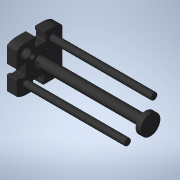
# Autodesk Inventor part: 537123 ADNGF-12-40-P-A---(KS)
Saved by Autodesk Inventor 2021 (Build 250183000, 183)
## iProperties
Created: 2025-06-05
Part Number: 537123 ADNGF-12-40-P-A---(KS)
Material: Generic
Catalog Web Link: www.cadenas.de
Description: ADNGF-(KS)-Compact cylinder - piston rod
Vendor: FESTO
Document SubType Name: Modeling
Designer: psAdmin
Manufacturer: FESTO
Mass: 6.99513 g
Surface Area: 56.7933 cm^2
Volume: 6.99513 cm^3
Density: 1 g/cm^3
Appearance: PSOLRGB-175-175-175
Category: PARTsolutions
Company: FESTO
Title: 537123 ADNGF-12-40-P-A---(KS)
Author: Cadenas PARTsolutions
Comments: Compact cylinder - piston rod
PSOL_IDENT_0: {$CADENAS_DATA/23d-libs/festo/parts/a/adngf/parts/adngf_ks.prj},219 {VTYP=3D},{NB=537123 ADNGF-12-40
PSOL_IDENT_1: -P-A---(KS)},{LINA=537123 ADNGF-12-40-P-A---(KS)},{NN=ADNGF-(KS)},{DATE=02.05.2022 12:53:58},{GEOMDA
PSOL_IDENT_2: TE=02.05.2022 12:53:00},{VERSION=},{LINEID=5510},{WBVAR=HUB,DF,S2S20},{WBNUMERIC=HUB}  {NB=537123 AD
PSOL_IDENT_3: NGF-12-40-P-A---(KS)},{LINA=537123 ADNGF-12-40-P-A---(KS)},{KT=ADNGF-12},{TNR=537123},{AUSF=ADNGF-12
PSOL_IDENT_4: },{HUB1=1.000},{HUB2=200.000},{KDM=12},{HUB=40},{TH=I},{THC='A','I'},{DF=P},{GA=A},{Q=-},{S2S20=-},{
PSOL_IDENT_5: K2=0},{K5=-},{K8=0},{K10=-},{S1=-},{TT=-},{R8=-},{A=10.000},{A1=0.000},{AF=8.000},{AF1=0.000},{AF2=8
PSOL_IDENT_6: .000},{AF3=0.000},{AF5=0.000},{AF7=0.000},{D8=0.000},{D9=0.000},{KF=M3},{KFN=3.000},{KF1=-},{KF1C=0.
PSOL_IDENT_7: 0000},{KF2=-},{KF2C=0.0000},{KF3=M3},{KF3C=3.0000},{KF5=-},{KF5N=0},{KF7=-},{KF7N=0},{KK=M5},{KKN=5}
PSOL_IDENT_8: ,{KKP=0.80},{KK1=-},{KK1N=0.0000},{KK1P=0.00},{L2=35.000},{L8=0.000},{MM=6.000},{MM1=0.000},{PL=6.00
PSOL_IDENT_9: 0},{SF=5},{SF1=0},{SF3=5.5},{WH1=4.200},{WH3=0.000},{WL=2.700},{WL1=0.000},{ZM=44.500},{ZM2=0.000},{
PSOL_IDENT_10: S2N=},{KKC3=3.800},{KKF2=0.400},{KKD5=0.900},{KKE2=20.000},{K5C3=0},{K5F2=0},{K5D5=0},{KK1C3=0.000},
PSOL_IDENT_11: {KK1F2=0.000},{KK1D5=0.000},{KK1E2=0.000},{ZA=35.000},{L100S1=0.000},{L101S1=0.000},{L102S1=0.000},{
PSOL_IDENT_12: L103S1=0.000},{D100S1=0.000},{L100=0.400},{L101=1.500},{L102=8.000},{L103=11.000},{D100=3.300},{L100
PSOL_IDENT_13: Q=0.400},{L101Q=1.500},{L101K5=1.500},{L102Q=8.000},{L103Q=11.000},{D100Q=3.300},{L100S1K5=0.000},{L
PSOL_IDENT_14: 101S1K5=0.000},{L102S1K5=0.000},{L103S1K5=0.000},{D100S1K5=0.000},{VERS=1},{WHX=4.2},{D20=0.000},{XF
PSOL_IDENT_15: 31=3.000},{B31=2.700},{WH=4.2},{DFALG='P'},{ZB=39.200},{ZB2=0.000},{W2=46.000},{W3=6.000},{W4=0.000}
PSOL_IDENT_16: ,{W5=0.000}
NB: 537123 ADNGF-12-40-P-A---(KS)
NN: ADNGF-(KS)
NT: Compact cylinder - piston rod
NBSYN: $TNR. $AUSF.-$HUB.-$DF.-$GA.$S2N.---(KS)
LINA: 537123 ADNGF-12-40-P-A---(KS)
CATALOG: Festo
TNR: 537123
AUSF: ADNGF-12
KDM: 12
HUB: 40
TH: I
DF: P
GA: A
Q: -
S2S20: -
K2: 0
K5: -
K8: 0
K10: -
S1: -
TT: -
R8: -
A: 10
A1: 0
AF: 8
AF1: 0
AF2: 8
AF3: 0
AF5: 0
AF7: 0
D8: 0
D9: 0
KF: M3
KF1: -
KF2: -
KF3: M3
KF5: -
KF7: -
KK: M5
KK1: -
L2: 35
L8: 0
MM: 6
MM1: 0
PL: 6
SF: 5
SF1: 0
SF3: 5.5
WH1: 4.2
WH3: 0
WL: 2.7
WL1: 0
ZM: 44.5
ZM2: 0
ZA: 35
L101K5: 1.5
D20: 0
XF31: 3
B31: 2.7
ZB: 39.2
ZB2: 0
W2: 46
W3: 6
W4: 0
W5: 0
SUPPLIER: FESTO
ARTICLENO: 537123 ADNGF-12-40-P-A---(KS)
BOMINFO: 537123 ADNGF-12-40-P-A---(KS)
CREATOR: CADENAS GmbH
Autodesk Inventor part; units mm, degrees
sketch "Sketch_1" plane through (0, 0, 0) normal (0, 0, 1) x (1, 0, 0)
  line L0 (63, 0) -> (-4.2, 0)
  line L1 (-4.2, 0) -> (-4.2, 3)
  line L2 (-4.2, 3) -> (63, 3)
  line L3 (63, 3) -> (63, 0)
  line L4 (63, 0) -> (-4.2, 0)
  constraints: 10 end point
revolve "Revolution1" add sketch "Sketch_1" angle 360 about axis through (63, 0, 0) along (1, 0, 0)
sketch "Sketch_11" plane through (0, 0, 0) normal (0, 0, 1) x (1, 0, 0)
  line L0 (63, 0) -> (60, 0)
  line L1 (60, 0) -> (60, 6)
  line L2 (60, 6) -> (63, 6)
  line L3 (63, 6) -> (63, 0)
  line L4 (63, 0) -> (60, 0)
  constraints: 10 end point
revolve "Revolution2" add sketch "Sketch_11" angle 360 about axis through (63, 0, 0) along (1, 0, 0)
sketch "Sketch_2" plane through (0, 0, 0) normal (0, 1, 0) x (-1, 0, 0)
  line L0 (23.4, 10.5) -> (-3.1188, 10.5)
  line L1 (-3.1188, 10.5) -> (1.5, 2.5)
  line L2 (1.5, 2.5) -> (4.2, 2.5)
  line L3 (4.2, 2.5) -> (4.2, 7.5)
  line L4 (4.2, 7.5) -> (19.2, 7.5)
  line L5 (19.2, 7.5) -> (19.2, -7.5)
  line L6 (19.2, -7.5) -> (4.2, -7.5)
  line L7 (4.2, -7.5) -> (4.2, -2.5)
  line L8 (4.2, -2.5) -> (1.5, -2.5)
  line L9 (1.5, -2.5) -> (-3.1188, -10.5)
  line L10 (-3.1188, -10.5) -> (23.4, -10.5)
  line L11 (23.4, -10.5) -> (23.4, 10.5)
  constraints: 24 end point
extrude "Extrusion1" cut sketch "Sketch_2" along normal mid plane 12
sketch "Sketch_5" plane through (-4.2, 0, 0) normal (1, 0, 0) x (0, 0, -1)
  arc A0 (-13.75, 2.5) -> (-13.35, 2.1) centre (-13.35, 2.5) ccw
  line L0 (-13.35, 2.1) -> (-11.9, 2.1)
  arc A1 (-11.9, 2.1) -> (-11.7, 2.3) centre (-11.9, 2.3) ccw
  line L1 (-11.7, 2.3) -> (-11.7, 2.6)
  arc A2 (-11.5, 2.8) -> (-11.7, 2.6) centre (-11.5, 2.6) ccw
  line L2 (-11.5, 2.8) -> (-8.7, 2.8)
  arc A3 (-8.3, 2.4) -> (-8.7, 2.8) centre (-8.7, 2.4) ccw
  line L3 (-8.3, 2.4) -> (-8.3, -3.6)
  arc A4 (-8.7, -4) -> (-8.3, -3.6) centre (-8.7, -3.6) ccw
  line L4 (-8.7, -4) -> (-11.5, -4)
  arc A5 (-11.7, -3.8) -> (-11.5, -4) centre (-11.5, -3.8) ccw
  line L5 (-11.7, -3.8) -> (-11.7, -3.5)
  arc A6 (-11.7, -3.5) -> (-11.9, -3.3) centre (-11.9, -3.5) ccw
  line L6 (-11.9, -3.3) -> (-13.35, -3.3)
  arc A7 (-13.35, -3.3) -> (-13.75, -3.7) centre (-13.35, -3.7) ccw
  line L7 (-13.75, -3.7) -> (-13.75, -11.5793)
  arc A8 (-13.75, -11.5793) -> (-13.3272, -12.3141) centre (-12.9, -11.5793) ccw
  arc A9 (-13.3272, -12.3141) -> (-8, -13.75) centre (-8, -3.15) ccw
  line L8 (-8, -13.75) -> (-3.7, -13.75)
  arc A10 (-3.7, -13.75) -> (-3.3, -13.35) centre (-3.7, -13.35) ccw
  line L9 (-3.3, -13.35) -> (-3.3, -11.9)
  arc A11 (-3.3, -11.9) -> (-3.5, -11.7) centre (-3.5, -11.9) ccw
  line L10 (-3.5, -11.7) -> (-3.8, -11.7)
  arc A12 (-4, -11.5) -> (-3.8, -11.7) centre (-3.8, -11.5) ccw
  line L11 (-4, -11.5) -> (-4, -8.7)
  arc A13 (-3.6, -8.3) -> (-4, -8.7) centre (-3.6, -8.7) ccw
  line L12 (-3.6, -8.3) -> (2.4, -8.3)
  arc A14 (2.8, -8.7) -> (2.4, -8.3) centre (2.4, -8.7) ccw
  line L13 (2.8, -8.7) -> (2.8, -11.5)
  arc A15 (2.6, -11.7) -> (2.8, -11.5) centre (2.6, -11.5) ccw
  line L14 (2.6, -11.7) -> (2.3, -11.7)
  arc A16 (2.3, -11.7) -> (2.1, -11.9) centre (2.3, -11.9) ccw
  line L15 (2.1, -11.9) -> (2.1, -13.35)
  arc A17 (2.1, -13.35) -> (2.5, -13.75) centre (2.5, -13.35) ccw
  line L16 (2.5, -13.75) -> (8, -13.75)
  arc A18 (8, -13.75) -> (13.3272, -12.3141) centre (8, -3.15) ccw
  arc A19 (13.3272, -12.3141) -> (13.75, -11.5793) centre (12.9, -11.5793) ccw
  line L17 (13.75, -11.5793) -> (13.75, 11.5793)
  arc A20 (13.75, 11.5793) -> (13.3272, 12.3141) centre (12.9, 11.5793) ccw
  arc A21 (13.3272, 12.3141) -> (8, 13.75) centre (8, 3.15) ccw
  line L18 (8, 13.75) -> (3.7, 13.75)
  arc A22 (3.7, 13.75) -> (3.3, 13.35) centre (3.7, 13.35) ccw
  line L19 (3.3, 13.35) -> (3.3, 11.9)
  arc A23 (3.3, 11.9) -> (3.5, 11.7) centre (3.5, 11.9) ccw
  line L20 (3.5, 11.7) -> (3.8, 11.7)
  arc A24 (4, 11.5) -> (3.8, 11.7) centre (3.8, 11.5) ccw
  line L21 (4, 11.5) -> (4, 8.7)
  arc A25 (3.6, 8.3) -> (4, 8.7) centre (3.6, 8.7) ccw
  line L22 (3.6, 8.3) -> (-2.4, 8.3)
  arc A26 (-2.8, 8.7) -> (-2.4, 8.3) centre (-2.4, 8.7) ccw
  line L23 (-2.8, 8.7) -> (-2.8, 11.5)
  arc A27 (-2.6, 11.7) -> (-2.8, 11.5) centre (-2.6, 11.5) ccw
  line L24 (-2.6, 11.7) -> (-2.3, 11.7)
  arc A28 (-2.3, 11.7) -> (-2.1, 11.9) centre (-2.3, 11.9) ccw
  line L25 (-2.1, 11.9) -> (-2.1, 13.35)
  arc A29 (-2.1, 13.35) -> (-2.5, 13.75) centre (-2.5, 13.35) ccw
  line L26 (-2.5, 13.75) -> (-8, 13.75)
  arc A30 (-8, 13.75) -> (-13.3272, 12.3141) centre (-8, 3.15) ccw
  arc A31 (-13.3272, 12.3141) -> (-13.75, 11.5793) centre (-12.9, 11.5793) ccw
  line L27 (-13.75, 11.5793) -> (-13.75, 2.5)
  circle A32 centre (8, -8) radius 3
  circle A33 centre (4.2426, -4.2426) radius 1.5
  circle A34 centre (-4.2426, 4.2426) radius 1.5
  circle A35 centre (-8, 8) radius 3
  constraints: 64 point on circle, 56 end point, 36 centre point
extrude "Extrusion2" add sketch "Sketch_5" against normal blind 6
sketch "Sketch_6" plane through (0, 0, 0) normal (0, 0, 1) x (1, 0, 0)
  line L0 (-7.634, 0) -> (-10.2, 0)
  line L1 (-10.2, 0) -> (-10.2, 3)
  line L2 (-10.2, 3) -> (-6.8, 3)
  line L3 (-6.8, 3) -> (-6.8, 2.75)
  line L4 (-6.8, 2.75) -> (-9.5, 2.75)
  arc A0 (-9.5, 2.75) -> (-9.8, 2.45) centre (-9.5, 2.45) ccw
  line L5 (-9.8, 2.45) -> (-9.8, 1.45)
  line L6 (-9.8, 1.45) -> (-9.6, 1.25)
  line L7 (-9.6, 1.25) -> (-8.3557, 1.25)
  line L8 (-8.3557, 1.25) -> (-7.634, 0)
  line L9 (-7.634, 0) -> (-10.2, 0)
  constraints: 20 end point, 2 point on circle, 1 centre point
revolve "Revolution3" cut sketch "Sketch_6" angle 360 about axis through (-7.634, 0, 0) along (1, 0, 0)
sketch "Sketch_7" plane through (0, 0, 0) normal (0, 0.7071068, 0.7071068) x (1, 0, 0)
  line L0 (-4.2, 6) -> (-10.2, 6)
  line L1 (-10.2, 6) -> (-10.2, 7.5)
  line L2 (-10.2, 7.5) -> (-9.9295, 7.2295)
  line L3 (-9.9295, 7.2295) -> (-4.4705, 7.2295)
  line L4 (-4.4705, 7.2295) -> (-4.2, 7.5)
  line L5 (-4.2, 7.5) -> (-4.2, 6)
  line L6 (-4.2, 6) -> (-10.2, 6)
  constraints: 14 end point
revolve "Revolution4" cut sketch "Sketch_7" angle 360 about axis through (-4.2, 4.2426, -4.2426) along (1, 0, 0)
thread "Thread1" size "M3x0.5" class "6H" standard "ISO Metric profile" full length
sketch "Sketch_8" plane through (0, 0, 0) normal (0, 0.7071068, 0.7071068) x (1, 0, 0)
  line L0 (-4.2, -6) -> (-10.2, -6)
  line L1 (-10.2, -6) -> (-10.2, -4.5)
  line L2 (-10.2, -4.5) -> (-9.9295, -4.7705)
  line L3 (-9.9295, -4.7705) -> (-4.4705, -4.7705)
  line L4 (-4.4705, -4.7705) -> (-4.2, -4.5)
  line L5 (-4.2, -4.5) -> (-4.2, -6)
  line L6 (-4.2, -6) -> (-10.2, -6)
  constraints: 14 end point
revolve "Revolution5" cut sketch "Sketch_8" angle 360 about axis through (-4.2, -4.2426, 4.2426) along (1, 0, 0)
thread "Thread2" size "M3x0.5" class "6H" standard "ISO Metric profile" full length
sketch "Sketch_9" plane through (0, 0, 0) normal (0, 0.7071068, 0.7071068) x (1, 0, 0)
  line L0 (-10.19, 11.3137) -> (-10.7, 11.3137)
  line L1 (-10.7, 11.3137) -> (-10.7, 13.6137)
  line L2 (-10.7, 13.6137) -> (-8.2, 13.6137)
  line L3 (-8.2, 13.6137) -> (-8.2, 13.2137)
  line L4 (-8.2, 13.2137) -> (-9.99, 13.2137)
  arc A0 (-9.99, 13.2137) -> (-10.19, 13.0137) centre (-9.99, 13.0137) ccw
  line L5 (-10.19, 13.0137) -> (-10.19, 11.3137)
  line L6 (-10.19, 11.3137) -> (-10.7, 11.3137)
  constraints: 14 end point, 2 point on circle, 1 centre point
revolve "Revolution6" cut sketch "Sketch_9" angle 360 about axis through (-10.19, 8, -8) along (1, 0, 0)
sketch "Sketch_13" plane through (0, 0, 0) normal (0, 0.7071068, 0.7071068) x (1, 0, 0)
  line L0 (-10.19, -11.3137) -> (-10.7, -11.3137)
  line L1 (-10.7, -11.3137) -> (-10.7, -9.0137)
  line L2 (-10.7, -9.0137) -> (-8.2, -9.0137)
  line L3 (-8.2, -9.0137) -> (-8.2, -9.4137)
  line L4 (-8.2, -9.4137) -> (-9.99, -9.4137)
  arc A0 (-9.99, -9.4137) -> (-10.19, -9.6137) centre (-9.99, -9.6137) ccw
  line L5 (-10.19, -9.6137) -> (-10.19, -11.3137)
  line L6 (-10.19, -11.3137) -> (-10.7, -11.3137)
  constraints: 14 end point, 2 point on circle, 1 centre point
revolve "Revolution7" cut sketch "Sketch_13" angle 360 about axis through (-10.19, -8, 8) along (1, 0, 0)
sketch "Sketch_15" plane through (-9.8, 0, 0) normal (1, 0, 0) x (0, 0, -1)
  line L0 (-1.25, -0.7217) -> (0, -1.4434)
  line L1 (0, -1.4434) -> (1.25, -0.7217)
  line L2 (1.25, -0.7217) -> (1.25, 0.7217)
  line L3 (1.25, 0.7217) -> (0, 1.4434)
  line L4 (0, 1.4434) -> (-1.25, 0.7217)
  line L5 (-1.25, 0.7217) -> (-1.25, -0.7217)
  constraints: 12 end point
extrude "Extrusion3" cut sketch "Sketch_15" along normal blind 1.3
sketch "Sketch_22" plane through (0, 0, 0) normal (0, 0.7071068, 0.7071068) x (1, 0, 0)
  line L0 (57.2, 11.3137) -> (-4.2, 11.3137)
  line L1 (-4.2, 11.3137) -> (-4.2, 13.3137)
  line L2 (-4.2, 13.3137) -> (57, 13.3137)
  line L3 (57, 13.3137) -> (57.2, 13.2601)
  line L4 (57.2, 13.2601) -> (57.2, 11.3137)
  line L5 (57.2, 11.3137) -> (-4.2, 11.3137)
  constraints: 12 end point
revolve "Revolution8" add sketch "Sketch_22" angle 360 about axis through (57.2, 8, -8) along (1, 0, 0)
sketch "Sketch_23" plane through (0, 0, 0) normal (0, 0.7071068, 0.7071068) x (1, 0, 0)
  line L0 (57.2, -11.3137) -> (-4.2, -11.3137)
  line L1 (-4.2, -11.3137) -> (-4.2, -9.3137)
  line L2 (-4.2, -9.3137) -> (57, -9.3137)
  line L3 (57, -9.3137) -> (57.2, -9.3673)
  line L4 (57.2, -9.3673) -> (57.2, -11.3137)
  line L5 (57.2, -11.3137) -> (-4.2, -11.3137)
  constraints: 12 end point
revolve "Revolution9" add sketch "Sketch_23" angle 360 about axis through (57.2, -8, 8) along (1, 0, 0)
sketch "Sketch_10" plane through (-10.19, -8, 8) normal (-1, 0, 0) x (0, 0.7071068, -0.7071068)
  line L0 (-0.75, -0.433) -> (0, -0.866)
  line L1 (0, -0.866) -> (0.75, -0.433)
  line L2 (0.75, -0.433) -> (0.75, 0.433)
  line L3 (0.75, 0.433) -> (0, 0.866)
  line L4 (0, 0.866) -> (-0.75, 0.433)
  line L5 (-0.75, 0.433) -> (-0.75, -0.433)
  constraints: 12 end point
extrude "Extrusion4" cut sketch "Sketch_10" against normal blind 1
sketch "Sketch_14" plane through (-10.19, 8, -8) normal (-1, 0, 0) x (0, 0.7071068, -0.7071068)
  line L0 (-0.75, -0.433) -> (0, -0.866)
  line L1 (0, -0.866) -> (0.75, -0.433)
  line L2 (0.75, -0.433) -> (0.75, 0.433)
  line L3 (0.75, 0.433) -> (0, 0.866)
  line L4 (0, 0.866) -> (-0.75, 0.433)
  line L5 (-0.75, 0.433) -> (-0.75, -0.433)
  constraints: 12 end point
extrude "Extrusion5" cut sketch "Sketch_14" against normal blind 1
ref_plane "PISTON_XY" through (63, 0, 0) normal (1, 0, 0) x (0, 0, -1)
ref_plane "PISTON_YZ" through (63, 0, 0) normal (0, 0, -1) x (0, 1, 0)
ref_plane "PISTON_ZX" through (63, 0, 0) normal (0, 1, 0) x (1, 0, 0)
body "Solid1"
